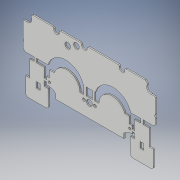
# Autodesk Inventor part: Controller_PCB_shape
Saved by Autodesk Inventor 2019 (Build 230136000, 136)
## iProperties
Created: 2019-05-16
Part Number: Controller_PCB_shape
Material: Generic
Document SubType Name: Modeling
Designer: cutla
Density: 1 g/cm^3
Appearance: Default
Author: cutla
Autodesk Inventor part; units mm, degrees
ref_plane "YZ Plane" through (0, 0, 0) normal (1, 0, 0) x (0, 1, 0)
ref_plane "XZ Plane" through (0, 0, 0) normal (0, 1, 0) x (-1, 0, 0)
ref_plane "XY Plane" through (0, 0, 0) normal (0, 0, 1) x (1, 0, 0)
sketch "Sketch1" plane through (0, 0, 0) normal (0, 0, 1) x (1, 0, 0)
  arc A0 (-3.7267, -16.0592) -> (-37.2524, -16.0592) centre (-20.4895, -21.1986) ccw
  line L0 (54.6611, 17.1124) -> (56.1788, 15.6393)
  arc A1 (40.8188, -16.0592) -> (7.4463, -16.0592) centre (24.1326, -21.0878) ccw
  line L1 (64.3275, -14.0592) -> (64.3275, -13.3371)
  line L2 (-60.6725, -12.69) -> (-60.6725, -14.0592)
  line L3 (-58.6725, -16.0592) -> (-58.1701, -16.0592)
  arc A2 (-57.4367, 9.2999) -> (-52.7991, 14.9932) centre (-56.4132, 13.2017) ccw
  arc A3 (56.3395, 14.4066) -> (60.3697, 8.5836) centre (59.6697, 12.4053) ccw
  line L4 (-52.1594, 16.9218) -> (-52.7531, 15.9643)
  line L5 (-57.4367, 9.2999) -> (-59.6725, 9.2999)
  line L6 (60.3697, 8.5836) -> (63.3275, 8.5836)
  line L7 (-60.6725, -14.0592) -> (-58.6725, -16.0592)
  line L8 (62.3275, -16.0592) -> (64.3275, -14.0592)
  arc A4 (-59.6725, 9.2999) -> (-60.6725, 8.2999) centre (-59.6725, 8.2999) ccw
  arc A5 (-52.7531, 15.9643) -> (-52.7991, 14.9932) centre (-51.9032, 15.4374) ccw
  arc A6 (-51.3095, 17.3948) -> (-52.1594, 16.9218) centre (-51.3095, 16.3948) ccw
  arc A7 (54.6611, 17.1124) -> (53.9646, 17.3948) centre (53.9646, 16.3948) ccw
  arc A8 (56.3395, 14.4066) -> (56.1788, 15.6393) centre (55.4824, 14.9217) ccw
  arc A9 (64.3275, 7.5836) -> (63.3275, 8.5836) centre (63.3275, 7.5836) ccw
  circle A10 centre (-10.3875, 12.8711) radius 2.6974
  circle A11 centre (-18.5554, 9.007) radius 2.6974
  arc A12 (-31.6739, 16.1713) -> (-26.4156, 16.1713) centre (-29.0448, 15.5685) ccw
  arc A13 (-5.4771, 16.2784) -> (-0.119, 16.2784) centre (-2.798, 15.9643) ccw
  arc A14 (30.0707, 16.1713) -> (35.329, 16.1713) centre (32.6999, 15.5685) ccw
  line L9 (-51.3095, 17.3948) -> (-32.6487, 17.3948)
  line L10 (-25.4409, 17.3948) -> (-6.4703, 17.3948)
  line L11 (0.8742, 17.3948) -> (29.096, 17.3948)
  line L12 (36.3037, 17.3948) -> (53.9646, 17.3948)
  arc A15 (-31.6739, 16.1713) -> (-32.6487, 17.3948) centre (-32.6487, 16.3948) ccw
  arc A16 (-25.4409, 17.3948) -> (-26.4156, 16.1713) centre (-25.4409, 16.3948) ccw
  arc A17 (-5.4771, 16.2784) -> (-6.4703, 17.3948) centre (-6.4703, 16.3948) ccw
  arc A18 (0.8742, 17.3948) -> (-0.119, 16.2784) centre (0.8742, 16.3948) ccw
  arc A19 (36.3037, 17.3948) -> (35.329, 16.1713) centre (36.3037, 16.3948) ccw
  arc A20 (30.0707, 16.1713) -> (29.096, 17.3948) centre (29.096, 16.3948) ccw
  arc A21 (-60.3022, -8.5391) -> (-60.3022, -6.3973) centre (-61.1704, -7.4682) ccw
  arc A22 (63.8977, -6.3786) -> (63.8977, -8.5579) centre (64.6538, -7.4682) ccw
  line L13 (-60.6725, 8.2999) -> (-60.6725, -5.6205)
  line L14 (-60.6725, -9.3159) -> (-60.6725, -12.69)
  line L15 (64.3275, 7.5836) -> (64.3275, -5.5571)
  line L16 (64.3275, -9.3794) -> (64.3275, -13.3371)
  arc A23 (63.8977, -6.3786) -> (64.3275, -5.5571) centre (63.3275, -5.5571) ccw
  arc A24 (64.3275, -9.3794) -> (63.8977, -8.5579) centre (63.3275, -9.3794) ccw
  arc A25 (-60.6725, -5.6205) -> (-60.3022, -6.3973) centre (-59.6725, -5.6205) ccw
  arc A26 (-60.3022, -8.5391) -> (-60.6725, -9.3159) centre (-59.6725, -9.3159) ccw
  line L17 (34.4431, -35.9938) -> (34.4431, -40.4667)
  line L18 (34.4431, -40.4667) -> (-29.9275, -40.4667)
  line L19 (-29.9275, -40.4667) -> (-29.9275, -35.9938)
  arc A27 (42.235, -32.8398) -> (34.4431, -35.9938) centre (41.595, -42.4607) ccw
  arc A28 (-29.9275, -35.9938) -> (-38.265, -32.8398) centre (-37.0762, -42.2942) ccw
  line L20 (42.235, -25.9841) -> (39.4133, -25.9841)
  line L21 (39.4133, -25.9841) -> (39.4133, -19.5932)
  line L22 (39.4133, -19.5932) -> (35.9618, -19.5932)
  arc A29 (35.2614, -19.5932) -> (10.8448, -23.4926) centre (23.4033, -23.7357) ccw
  arc A30 (-6.9895, -23.4926) -> (-31.2991, -19.5932) centre (-19.4667, -23.5527) ccw
  line L23 (35.9618, -19.5932) -> (35.2614, -19.5932)
  line L24 (-38.265, -25.9841) -> (-35.7909, -25.9841)
  line L25 (-35.7909, -25.9841) -> (-35.7909, -19.5932)
  line L26 (-35.7909, -19.5932) -> (-31.2991, -19.5932)
  circle A31 centre (39.9237, -29.5672) radius 1.1216
  circle A32 centre (-35.7909, -29.5672) radius 1.1216
  circle A33 centre (1.9276, -27.6516) radius 2.7746
  circle A34 centre (7.1158, -27.4394) radius 1.3953
  circle A35 centre (-3.253, -27.4394) radius 1.3878
  line L27 (40.6807, -35.3184) -> (40.6807, -49.6691)
  line L28 (43.1807, -52.1691) -> (59.6317, -52.1691)
  line L29 (62.1317, -49.6691) -> (62.1317, -35.3184)
  line L30 (58.1708, -19.7658) -> (58.1708, -35.3184)
  arc A36 (59.6317, -52.1691) -> (62.1317, -49.6691) centre (59.6317, -49.6691) ccw
  arc A37 (40.6807, -49.6691) -> (43.1807, -52.1691) centre (43.1807, -49.6691) ccw
  line L31 (62.1317, -35.3184) -> (58.1708, -35.3184)
  line L32 (44.515, -35.3184) -> (40.6807, -35.3184)
  line L33 (62.1317, -35.3184) -> (58.1708, -35.3184)
  line L34 (44.515, -35.3184) -> (40.6807, -35.3184)
  line L35 (53.2836, -40.5985) -> (49.6315, -40.5985)
  line L36 (49.6315, -40.5985) -> (49.6315, -35.1536)
  line L37 (49.6315, -35.1536) -> (53.2836, -35.1536)
  line L38 (53.2836, -35.1536) -> (53.2836, -40.5985)
  line L39 (-58.1639, -35.1992) -> (-58.1639, -49.55)
  line L40 (-55.6639, -52.05) -> (-39.2129, -52.05)
  line L41 (-36.7129, -49.55) -> (-36.7129, -35.1992)
  line L42 (-54.3296, -35.1992) -> (-54.3296, -19.6467)
  arc A38 (-39.2129, -52.05) -> (-36.7129, -49.55) centre (-39.2129, -49.55) ccw
  arc A39 (-58.1639, -49.55) -> (-55.6639, -52.05) centre (-55.6639, -49.55) ccw
  line L43 (-36.7129, -35.1992) -> (-40.6737, -35.1992)
  line L44 (-54.3296, -35.1992) -> (-58.1639, -35.1992)
  line L45 (-36.7129, -35.1992) -> (-40.6737, -35.1992)
  line L46 (-54.3296, -35.1992) -> (-58.1639, -35.1992)
  line L47 (-44.429, -40.4793) -> (-48.0811, -40.4793)
  line L48 (-48.0811, -40.4793) -> (-48.0811, -35.0344)
  line L49 (-48.0811, -35.0344) -> (-44.429, -35.0344)
  line L50 (-44.429, -35.0344) -> (-44.429, -40.4793)
  line L51 (-48.0811, -16.0592) -> (-48.0811, -19.6467)
  line L52 (-50.0811, -19.6467) -> (-50.0811, -16.0592)
  line L53 (-40.6737, -28.6265) -> (-38.265, -28.6265)
  line L54 (-38.265, -30.6265) -> (-40.6737, -30.6265)
  line L55 (-1.253, -16.0592) -> (-1.253, -23.4926)
  line L56 (-3.253, -23.4926) -> (-3.253, -16.0592)
  line L57 (6.8345, -16.0592) -> (6.8345, -23.4926)
  line L58 (4.8345, -23.4926) -> (4.8345, -16.0592)
  line L59 (42.235, -28.8272) -> (44.515, -28.8272)
  line L60 (44.515, -30.8272) -> (42.235, -30.8272)
  line L61 (52.4918, -16.0592) -> (52.4918, -19.7658)
  line L62 (50.4918, -19.7658) -> (50.4918, -16.0592)
  line L63 (-54.3296, -19.6467) -> (-50.0811, -19.6467)
  line L64 (-48.0811, -19.6467) -> (-40.6737, -19.6467)
  line L65 (-58.1701, -16.0592) -> (-50.0811, -16.0592)
  line L66 (-48.0811, -16.0592) -> (-37.2524, -16.0592)
  line L67 (-40.6737, -19.6467) -> (-40.6737, -28.6265)
  line L68 (-40.6737, -30.6265) -> (-40.6737, -35.1992)
  line L69 (-38.265, -32.8398) -> (-38.265, -30.6265)
  line L70 (-38.265, -28.6265) -> (-38.265, -25.9841)
  line L71 (-3.7267, -16.0592) -> (-3.253, -16.0592)
  line L72 (-1.253, -16.0592) -> (4.8345, -16.0592)
  line L73 (6.8345, -16.0592) -> (7.4463, -16.0592)
  line L74 (10.8448, -23.4926) -> (6.8345, -23.4926)
  line L75 (4.8345, -23.4926) -> (-1.253, -23.4926)
  line L76 (-3.253, -23.4926) -> (-6.9895, -23.4926)
  line L77 (42.235, -25.9841) -> (42.235, -28.8272)
  line L78 (42.235, -30.8272) -> (42.235, -32.8398)
  line L79 (44.515, -35.3184) -> (44.515, -30.8272)
  line L80 (44.515, -28.8272) -> (44.515, -19.7658)
  line L81 (40.8188, -16.0592) -> (50.4918, -16.0592)
  line L82 (52.4918, -16.0592) -> (62.3275, -16.0592)
  line L83 (44.515, -19.7658) -> (50.4918, -19.7658)
  line L84 (52.4918, -19.7658) -> (58.1708, -19.7658)
  point P0 (0, 0)
  point P1 (56.8058, 15.0308)
  point P2 (64.3275, -16.0592)
  point P3 (-60.6725, -16.0592)
  point P4 (-53.0682, 15.4561)
  point P5 (-31.0298, 17.3948)
  point P6 (-27.0597, 17.3948)
  point P7 (-5.0849, 17.3948)
  point P8 (-0.5112, 17.3948)
  point P9 (30.7148, 17.3948)
  point P10 (34.6849, 17.3948)
  point P11 (-60.6725, -8.7538)
  point P12 (-60.6725, -6.1827)
  point P13 (64.3275, -6.1827)
  point P14 (64.3275, -8.7538)
  constraints: 170 end point, 78 point on circle, 48 tangent, 40 centre point, 21 parallel, 15 equal radius, 15 point on line, 13 perpendicular, 10 horizontal, 5 vertical
extrude "Extrusion1" add sketch "Sketch1" along normal blind 1.2
body "Solid1"
